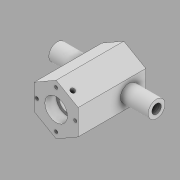
# Autodesk Inventor part: Válvula A01209499
Saved by Autodesk Inventor 2020 (Build 240168000, 168)
## iProperties
Created: 2019-10-23
Part Number: Válvula A01209499
Material: Genérico
Document SubType Name: Modeling
Designer: gerar
Density: 1 g/cm^3
Appearance: Valor por defecto
Author: Gerardo Naranjo
Autodesk Inventor part; units mm, degrees
ref_plane "YZ Plane" through (0, 0, 0) normal (1, 0, 0) x (0, 1, 0)
ref_plane "XZ Plane" through (0, 0, 0) normal (0, 1, 0) x (-1, 0, 0)
ref_plane "XY Plane" through (0, 0, 0) normal (0, 0, 1) x (1, 0, 0)
sketch "Boceto1" plane through (0, 0, 0) normal (0, 0, 1) x (1, 0, 0)
  circle A0 centre (0, 0) radius 28.575 construction
  line L0 (0, 28.575) -> (24.7467, 14.2875)
  line L1 (24.7467, 14.2875) -> (24.7467, -14.2875)
  line L2 (24.7467, -14.2875) -> (0, -28.575)
  line L3 (0, -28.575) -> (-24.7467, -14.2875)
  line L4 (-24.7467, -14.2875) -> (-24.7467, 14.2875)
  line L5 (-24.7467, 14.2875) -> (0, 28.575)
  circle A1 centre (0, 0) radius 21.59 construction
  dimension "d1" = 57.15
  dimension "d2" = 43.18
  constraints: 12 end point, 3 coincident, 1 centre point, 1 vertical alignment, 15 other
  measures "d2" diameter of A1
extrude "Hexagono" add sketch "Boceto1" along normal blind 76.2
sketch "Boceto2" plane through (0, 0, 76.2) normal (0, 0, 1) x (1, 0, 0)
  circle A0 centre (0, 0) radius 21.59 construction
  point P0 (0, 21.59)
  point P1 (21.59, 0)
  point P2 (-21.59, 0)
  point P3 (0, -21.59)
  dimension "d5" = 43.18
  constraints: 4 point on circle, 1 centre point, 1 coincident
  measures "d5" diameter of A0
hole "Tornillos" at (0, 21.59, 76.2) at (21.59, 0, 76.2) at (-21.59, 0, 76.2) at (0, -21.59, 76.2) direction (0, 0, -1) diameter 3.683 depth 14.224 tip angle 118 thread size "10-24 UNC" class "2B" standard "ANSI Unified Screw Threads"
sketch "Boceto3" plane through (0, 0, 0) normal (0, 0, -1) x (-1, 0, 0)
  circle A0 centre (0, 0) radius 19.05
  dimension "d13" = 38.1
  constraints: 1 centre point, 1 coincident
  measures "d13" diameter of A0
extrude "Extrusión2" cut sketch "Boceto3" against normal blind 38.1
sketch "Boceto5" plane through (0, 0, 76.2) normal (0, 0, 1) x (1, 0, 0)
  point P0 (0, 0)
  point P1 (0, 0)
  constraints: 1 coincident
hole "Agujero3" at (0, 0, 76.2) direction (0, 0, -1) diameter 19.05 depth 38.1 counterbore diameter 25.4 counterbore depth 12.7
chamfer "Chaflán2" distance 9.525 angle 45 1 edges at (0, 9.525, 38.1) measured on face at (0, 10.025, 38.1)
sketch "Boceto6" plane through (0, 0, 0) normal (1, 0, 0) x (0, 1, 0)
  line L0 (-14.2875, 0) -> (14.2875, 0) projected
  line L1 (-28.575, 0) -> (-28.575, 76.2) projected
  line L2 (28.575, 0) -> (28.575, 76.2) projected
  circle A0 centre (0, 19.05) radius 9.525
  point P0 (0, 0)
  dimension "d36" = 19.05
  dimension "d37" = 57.15
  dimension "d38" = 28.575
  dimension "d39" = 19.05
  constraints: 1 centre point, 1 coincident
  measures "d36" distance from line of L0 point (0, 19.05)
  measures "d37" distance between parallel lines of L1 L2
  measures "d38" distance from line of L2 point (0, 19.05)
  measures "d39" diameter of A0
extrude "Extrusión3" add sketch "Boceto6" along normal mid plane 111.76
sketch "Boceto7" plane through (55.88, 0, 19.05) normal (1, 0, 0) x (0, 0, -1)
  point P0 (19.05, 0)
  point P1 (0, 0)
hole "Agujero4" at (55.88, 0, 19.05) direction (-1, 0, 0) diameter 10.5918 end through all thread size "1/2-13 UNC" class "2B" standard "ANSI Unified Screw Threads"
sketch "Boceto8" plane through (0, 28.575, 76.2) normal (0.5, 0.8660254, 0) x (0.8660254, -0.5, 0)
  line L0 (28.575, 0) -> (0, 0) projected
  line L1 (42.8625, 76.2) -> (42.8625, 0) projected
  line L2 (-14.2875, 76.2) -> (-14.2875, 0) projected
  point P0 (14.2875, 76.2)
  point P1 (14.2875, 6.35)
  dimension "d49" = 6.35
  dimension "d50" = 57.15
  dimension "d51" = 28.575
  measures "d49" distance from line of L0 point (14.287, 6.35)
  measures "d50" distance between parallel lines of L1 L2
  measures "d51" distance from line of L2 point (14.287, 6.35)
hole "Agujero5" at (12.3733, 21.4312, 69.85) direction (-0.5, -0.8660254, 0) diameter 3.683 depth 14.9352 counterbore diameter 5.08 counterbore depth 9.525 thread size "10-24 UNC" class "2B" standard "ANSI Unified Screw Threads"
equation "\"d38\" = 0.5 * d37"
equation "\"d51\" = 0.5 * d50"
